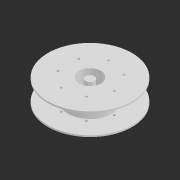
# Autodesk Inventor part: spool
Saved by Autodesk Inventor 2020.3 (Build 243373010, 373A)
## iProperties
Created: 2021-02-15
Part Number: spool
Material: Generic
Document SubType Name: Modeling
Designer: Melvin Strobl
Density: 1 g/cm^3
Appearance: Default
Mass: 165.518 g
Surface Area: 697.426 cm^2
Volume: 165.518 cm^3
Author: Melvin Strobl
Autodesk Inventor part; units mm, degrees
ref_plane "YZ Plane" through (0, 0, 0) normal (1, 0, 0) x (0, 1, 0)
ref_plane "XZ Plane" through (0, 0, 0) normal (0, 1, 0) x (-1, 0, 0)
ref_plane "XY Plane" through (0, 0, 0) normal (0, 0, 1) x (1, 0, 0)
sketch "Sketch1" plane through (0, 0, 0) normal (0, 1, 0) x (-1, 0, 0)
  circle A0 centre (0, 0) radius 52.5
  circle A1 centre (0, 0) radius 100
  circle A2 centre (0, 0) radius 26.2
  circle A3 centre (-57.5, 0) radius 3
  line L0 (140, 0) -> (-140, 0) projected
  circle A4 centre (-35.8507, -44.9553) radius 3
  circle A5 centre (12.795, -56.0584) radius 3
  circle A6 centre (51.8057, -24.9483) radius 3
  circle A7 centre (51.8057, 24.9483) radius 3
  circle A8 centre (12.795, 56.0584) radius 3
  circle A9 centre (-35.8507, 44.9553) radius 3
  line L1 (-10, -4.1421) -> (-10, 4.1421)
  line L2 (-10, 4.1421) -> (-4.1421, 10)
  line L3 (-4.1421, 10) -> (4.1421, 10)
  line L4 (4.1421, 10) -> (10, 4.1421)
  line L5 (10, 4.1421) -> (10, -4.1421)
  line L6 (10, -4.1421) -> (4.1421, -10)
  line L7 (4.1421, -10) -> (-4.1421, -10)
  line L8 (-4.1421, -10) -> (-10, -4.1421)
  line L9 (0, -140) -> (0, 140) projected
  dimension "d0" = 105
  dimension "d1" = 200
  dimension "d8" = 52.4
  dimension "d9" = 6
  dimension "d10" = 57.5
  dimension "d13" = 360
  dimension "d15" = 20
  constraints: 16 end point, 10 centre point, 4 coincident, 1 perpendicular, 1 point on line, 32 other
  measures "d0" diameter of A0
  measures "d1" diameter of A1
  measures "d8" diameter of A2
  measures "d9" diameter of A3
  measures "d10" distance of A3.centre point (0, 0)
  measures "d15" distance between parallel lines of L5 L1
extrude "Extrusion1" add sketch "Sketch1" along normal blind 3.75 contours L0 A1 L9 A0 | A0 L9 A1 L0 | A0 L0 A3 A1 L9 | L9 A1 L0 A3 A0
extrude "Extrusion2" add sketch "Sketch1" along normal blind 53 contours L0 A2 L9 A0 | A0 L9 A2 L0 | L9 A2 L0 A0 | A0 L0 A2 L9
extrude "Extrusion3" add sketch "Sketch1" against normal blind 3.75 from surface at 53 contours L0 A1 L9 A0 | A0 L9 A1 L0 | A0 L0 A3 A1 L9 | L9 A1 L0 A3 A0
extrude "Extrusion4" add sketch "Sketch1" along normal blind 50 contours L5 L6 L7 L9 L0 | L0 L9 L3 L4 L5 | L9 L0 L1 L2 L3 | L7 L8 L1 L0 L9
body "Solid1"
